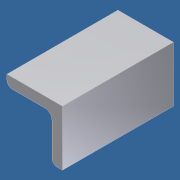
# Autodesk Inventor part: GE-12027-06
Saved by Autodesk Inventor 2012 (Build 160160000, 160)
## iProperties
Created: 2011-10-10
Part Number: GE-12027-06
Document SubType Name: Modeling
Designer: dfoster
Density: 1 g/cm^3
Description: Mounting Bracket
Material: Default
Title: Mounting Bracket
Author: dfoster
Autodesk Inventor part; units mm, degrees
ref_plane "YZ Plane" through (0, 0, 0) normal (1, 0, 0) x (0, 1, 0)
ref_plane "XZ Plane" through (0, 0, 0) normal (0, 1, 0) x (-1, 0, 0)
ref_plane "XY Plane" through (0, 0, 0) normal (0, 0, 1) x (1, 0, 0)
sketch "Sketch1" plane through (0, 0, 0) normal (0, 0, 1) x (1, 0, 0)
  line L0 (0, 0) -> (0, -25.4)
  line L1 (0, -25.4) -> (-2.3749, -25.4)
  line L2 (-4.7625, -23.0124) -> (-4.7625, -7.9375)
  line L3 (-7.9375, -4.7625) -> (-23.0124, -4.7625)
  line L4 (-25.4, -2.3749) -> (-25.4, 0)
  line L5 (-25.4, 0) -> (0, 0)
  arc A0 (-4.7625, -7.9375) -> (-7.9375, -4.7625) centre (-7.9375, -7.9375) ccw
  arc A1 (-25.4, -2.3749) -> (-23.0124, -4.7625) centre (-23.0124, -2.3749) ccw
  arc A2 (-4.7625, -23.0124) -> (-2.3749, -25.4) centre (-2.3749, -23.0124) ccw
  dimension "d2" = 25.4
  dimension "d3" = 4.7625
  dimension "d4" = 3.175
  dimension "d5" = 2.3876
  constraints: 12 end point, 6 point on circle, 6 tangent, 4 parallel, 3 centre point, 3 perpendicular, 1 equal radius, 1 vertical
  measures "d2" distance of L0.start L0.end
  measures "d3" distance between parallel lines of L2 L0
  measures "d4" radius of A0
  measures "d5" radius of A1
extrude "Extrusion1" add sketch "Sketch1" along normal blind 50.8
body "Solid1"
